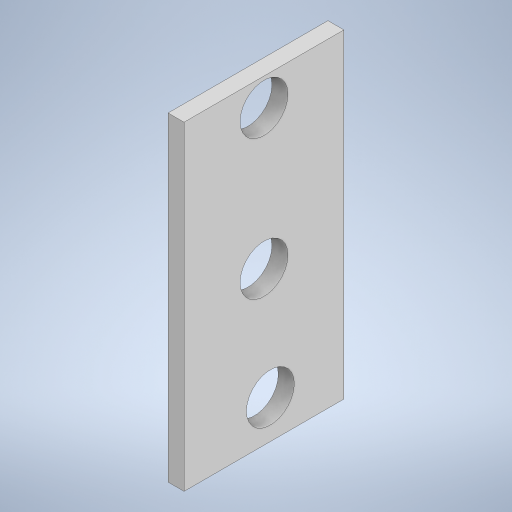
# Autodesk Inventor part: clamp
Saved by Autodesk Inventor 2023 (Build 270158000, 158)
## iProperties
Created: 2022-07-02
Part Number: clamp
Material: Generic
Document SubType Name: Modeling
Designer: anush
Density: 1 g/cm^3
Appearance: Default
Author: anush
Autodesk Inventor part; units mm, degrees
ref_plane "YZ Plane" through (0, 0, 0) normal (1, 0, 0) x (0, 1, 0)
ref_plane "XZ Plane" through (0, 0, 0) normal (0, 1, 0) x (-1, 0, 0)
ref_plane "XY Plane" through (0, 0, 0) normal (0, 0, 1) x (1, 0, 0)
sketch "Sketch1" plane through (0, 0, 0) normal (1, 0, 0) x (0, 1, 0)
  line L0 (11.2159, 27.719) -> (-8.7841, 27.719)
  line L1 (-8.7841, 27.719) -> (-8.7841, 17.719)
  line L2 (-8.7841, 17.719) -> (11.2159, 17.719)
  line L3 (11.2159, 17.719) -> (11.2159, 27.719)
  point P0 (0, 0)
  dimension "d0" = 20
  dimension "d1" = 10
  constraints: 8 end point, 2 parallel, 1 horizontal, 1 perpendicular
  measures "d0" distance of L2.end L1.end
  measures "d1" distance of L1.end L0.end
extrude "Extrusion1" add sketch "Sketch1" along normal blind 1
sketch "Sketch2" plane through (1, 0, 0) normal (1, 0, 0) x (0, 0, -1)
  circle A0 centre (-22.7194, 9.4904) radius 1.5
  circle A1 centre (-22.7194, 0.7743) radius 1.5
  circle A2 centre (-22.3212, -6.3933) radius 1.5
  point P0 (0, 0)
  dimension "d4" = 3
  dimension "d5" = 3
  dimension "d6" = 3
  constraints: 3 centre point
  measures "d4" diameter of A0
  measures "d5" diameter of A1
  measures "d6" diameter of A2
hole "Hole1" at (1, 9.4904, 22.7194) at (1, -6.3933, 22.3212) at (1, 0.7743, 22.7194) direction (-1, 0, 0) diameter 3 end through all
equation "\"d7\" = d6"
body "Solid1"
